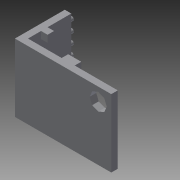
# Autodesk Inventor part: polyoctpart
Saved by Autodesk Inventor 2015 SP1 (Build 190203100, 203)
## iProperties
Created: 2015-04-18
Part Number: polyoctpart
Material: Generic
Document SubType Name: Modeling
Designer: Lab User
Density: 1 g/cm^3
Appearance: Default
Author: Lab User
Autodesk Inventor part; units mm, degrees
ref_plane "YZ Plane" through (0, 0, 0) normal (1, 0, 0) x (0, 1, 0)
ref_plane "XZ Plane" through (0, 0, 0) normal (0, 1, 0) x (-1, 0, 0)
ref_plane "XY Plane" through (0, 0, 0) normal (0, 0, 1) x (1, 0, 0)
sketch "Sketch1" plane through (0, 0, 0) normal (0, 0, 1) x (1, 0, 0)
  line L0 (0, 8.2967) -> (5.8666, 5.8666)
  line L1 (5.8666, 5.8666) -> (8.2967, 0)
  line L2 (8.2967, 0) -> (5.8666, -5.8666)
  line L3 (5.8666, -5.8666) -> (0, -8.2967)
  line L4 (0, -8.2967) -> (-5.8666, -5.8666)
  line L5 (-5.8666, -5.8666) -> (-8.2967, 0)
  line L6 (-8.2967, 0) -> (-5.8666, 5.8666)
  line L7 (-5.8666, 5.8666) -> (0, 8.2967)
  line L8 (-81.026, 12.7) -> (12.7, 12.7)
  line L9 (12.7, 12.7) -> (12.7, -53.34)
  line L10 (12.7, -53.34) -> (-81.026, -53.34)
  line L11 (-81.026, -53.34) -> (-81.026, 12.7)
  point P0 (0, 0)
  point P1 (0, 0)
  dimension "d0" = 6.35
  dimension "d1" = 12.7
  dimension "d2" = 12.7
  dimension "d3" = 53.34
  dimension "d4" = 93.726
  constraints: 24 end point, 2 parallel, 1 coincident, 1 horizontal, 1 perpendicular, 17 other
  measures "d0" distance of L1.end L2.end
  measures "d1" distance from line of L9 point (0, 0)
  measures "d2" distance from line of L8 point (0, 0)
  measures "d3" distance from line of L10 point (0, 0)
  measures "d4" distance between parallel lines of L11 L9
extrude "Extrusion1" add sketch "Sketch1" along normal blind 6.35
sketch "Sketch2" plane through (0, 0, 0) normal (0, 0, -1) x (-1, 0, 0)
  line L0 (81.026, -53.34) -> (-12.7, -53.34) projected
  line L1 (81.026, 12.7) -> (74.676, 12.7)
  line L2 (74.676, 12.7) -> (74.676, -53.34)
  line L3 (74.676, -53.34) -> (81.026, -53.34)
  line L4 (81.026, -53.34) -> (81.026, 12.7)
  point P0 (0, 0)
  dimension "d7" = 6.35
  constraints: 8 end point, 2 parallel, 1 horizontal, 1 perpendicular, 1 point on line
  measures "d7" distance between parallel lines of L4 L2
extrude "Extrusion2" add sketch "Sketch2" along normal blind 42.164
sketch "Sketch3" plane through (0, 0, -42.164) normal (0, 0, -1) x (-1, 0, 0)
  circle A0 centre (77.851, 5.08) radius 1.905
  circle A1 centre (77.851, -5.08) radius 1.905
  circle A2 centre (77.851, -15.24) radius 1.905
  circle A3 centre (77.851, -25.4) radius 1.905
  line L0 (81.026, -53.34) -> (81.026, 12.7) projected
  line L1 (81.026, 12.7) -> (74.676, 12.7) projected
  circle A4 centre (77.851, -35.56) radius 1.905
  circle A5 centre (77.851, -45.72) radius 1.905
  line L2 (74.676, -53.34) -> (81.026, -53.34) projected
  point P0 (0, 0)
  dimension "d10" = 3.81
  dimension "d11" = 3.175
  dimension "d12" = 7.62
  dimension "d13" = 3.81
  dimension "d14" = 3.175
  dimension "d15" = 10.16
  dimension "d16" = 3.81
  dimension "d17" = 10.16
  dimension "d18" = 3.175
  dimension "d19" = 3.81
  dimension "d20" = 3.175
  dimension "d21" = 10.16
  dimension "d26" = 3.81
  dimension "d27" = 3.175
  dimension "d28" = 3.81
  dimension "d29" = 10.16
  dimension "d30" = 3.175
  dimension "d31" = 7.62
  dimension "d43" = 10.16
  constraints: 6 centre point
  measures "d10" diameter of A0
  measures "d11" distance from line of A0.centre L0
  measures "d12" distance from line of L1 A0.centre
  measures "d13" diameter of A1
  measures "d14" distance from line of L0 A1.centre
  measures "d15" distance of A0.centre A1.centre
  measures "d16" diameter of A2
  measures "d17" distance of A1.centre A2.centre
  measures "d18" distance from line of L0 A2.centre
  measures "d19" diameter of A3
  measures "d20" distance from line of L0 A3.centre
  measures "d21" distance of A2.centre A3.centre
  measures "d26" diameter of A4
  measures "d27" distance from line of L0 A4.centre
  measures "d28" diameter of A5
  measures "d29" distance of A4.centre A5.centre
  measures "d30" distance from line of L0 A5.centre
  measures "d31" distance from line of L2 A5.centre
  measures "d43" distance of A3.centre A4.centre
extrude "Extrusion3" add sketch "Sketch3" along normal blind 3.81
sketch "Sketch4" plane through (0, 0, 0) normal (0, 0, -1) x (-1, 0, 0)
  line L0 (5.8666, 5.8666) -> (50.455, 5.8666)
  line L1 (74.676, 12.7) -> (-12.7, 12.7) projected
  line L2 (15.8582, 12.7) -> (28.5582, 12.7)
  line L3 (28.5582, 5.8666) -> (15.8582, 5.8666)
  line L4 (41.91, 12.7) -> (29.21, 12.7)
  line L5 (29.21, 12.7) -> (29.21, 5.8666)
  line L6 (29.21, 5.8666) -> (41.91, 5.8666)
  line L7 (41.91, 5.8666) -> (41.91, 12.7)
  line L8 (-12.7, 12.7) -> (-12.7, -53.34) projected
  point P0 (0, 0)
  dimension "d35" = 12.7
  dimension "d36" = 41.91
  constraints: 14 end point, 4 point on line, 3 horizontal, 3 parallel, 1 perpendicular
  measures "d35" distance between parallel lines of L7 L5
  measures "d36" distance between parallel lines of L8 L5
extrude "Extrusion4" add sketch "Sketch4" along normal blind 6.35
sketch "Sketch5" plane through (-74.676, -53.34, 0) normal (1, 0, 0) x (0, 0, -1)
  line L0 (0, 59.2066) -> (28.7051, 59.2066)
  line L1 (0, 59.2066) -> (6.35, 59.2066) projected
  line L2 (0, 66.04) -> (42.164, 66.04) projected
  line L3 (19.05, 59.2066) -> (12.7, 59.2066)
  line L4 (12.7, 59.2066) -> (12.7, 66.04)
  line L5 (12.7, 66.04) -> (19.05, 66.04)
  line L6 (19.05, 66.04) -> (19.05, 59.2066)
  line L7 (-6.35, 0) -> (-6.35, 66.04) projected
  point P0 (0, 53.34)
  dimension "d39" = 6.35
  dimension "d40" = 19.05
  constraints: 10 end point, 2 parallel, 2 point on line, 1 collinear, 1 horizontal, 1 perpendicular
  measures "d39" distance between parallel lines of L6 L4
  measures "d40" distance between parallel lines of L7 L4
extrude "Extrusion5" add sketch "Sketch5" along normal blind 6.35
body "Solid1"
